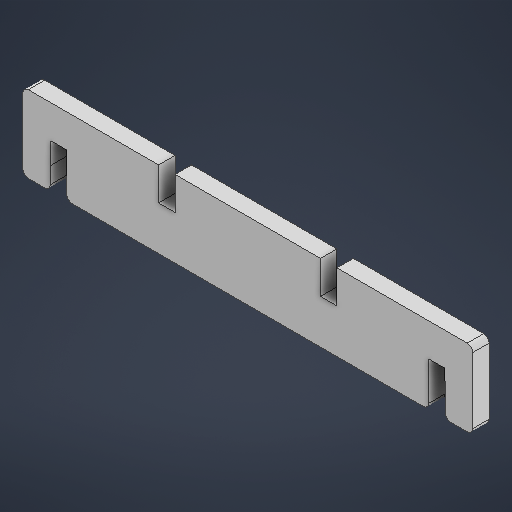
# Autodesk Inventor part: test
Saved by Autodesk Inventor 2025.3 (Build 293356030, 356C)
## iProperties
Created: 2025-10-02
Part Number: test
Material: 一般
Document SubType Name: Modeling
Designer: 陳泓任
Density: 1 g/cm^3
Appearance: 預設
Author: 陳泓任
Autodesk Inventor part; units mm, degrees
ref_plane "YZ Plane" through (0, 0, 0) normal (1, 0, 0) x (0, 1, 0)
ref_plane "XZ Plane" through (0, 0, 0) normal (0, 1, 0) x (-1, 0, 0)
ref_plane "XY Plane" through (0, 0, 0) normal (0, 0, 1) x (1, 0, 0)
sketch "草圖1" plane through (0, 0, 0) normal (0, 0, 1) x (1, 0, 0)
  line L0 (41, -6) -> (41, 6)
  line L1 (-41, 6) -> (-41, -6)
  line L2 (-40, -7) -> (-37, -7)
  line L3 (-32, -7) -> (32, -7)
  line L4 (37, -7) -> (40, -7)
  line L5 (0, 22.1211) -> (0, -32.4412) construction
  arc A0 (-40, 7) -> (-41, 6) centre (-40, 6) ccw
  arc A1 (-41, -6) -> (-40, -7) centre (-40, -6) ccw
  arc A2 (-37, -7) -> (-36, -6) centre (-37, -6) ccw
  arc A3 (-33, -6) -> (-32, -7) centre (-32, -6) ccw
  arc A4 (40, -7) -> (41, -6) centre (40, -6) ccw
  arc A5 (41, 6) -> (40, 7) centre (40, 6) ccw
  line L6 (-36, -6) -> (-36, 1) construction
  line L7 (-36, 1) -> (-33, 1) construction
  line L8 (-33, 1) -> (-33, -6)
  arc A6 (36, -6) -> (37, -7) centre (37, -6) ccw
  arc A7 (32, -7) -> (33, -6) centre (32, -6) ccw
  line L9 (36, -6) -> (36, 1) construction
  line L10 (36, 1) -> (33, 1) construction
  line L11 (33, 1) -> (33, -6)
  line L12 (-16.25, 7) -> (-16.25, 1)
  line L13 (-16.25, 1) -> (-13.25, 1)
  line L14 (-13.25, 1) -> (-13.25, 7)
  line L15 (-14.75, -1.2757) -> (-14.75, 3.2757) construction
  line L16 (16.25, 7) -> (16.25, 1)
  line L17 (16.25, 1) -> (13.25, 1)
  line L18 (13.25, 1) -> (13.25, 7)
  line L19 (-41, -7) -> (41, -7) construction
  line L20 (41, -7) -> (41, 7) construction
  line L21 (41, 7) -> (-41, 7) construction
  line L22 (-41, 7) -> (-41, -7) construction
  line L23 (-41, -7) -> (41, 7) construction
  line L24 (41, -7) -> (-41, 7) construction
  line L25 (-16.25, 7) -> (-40, 7)
  line L26 (40, 7) -> (16.25, 7)
  line L27 (13.25, 7) -> (-13.25, 7)
  line L28 (-36, -6) -> (-36, -3)
  line L29 (-35.9, 1) -> (-36, -3)
  line L30 (-35.9, 1) -> (-33, 1)
  line L31 (35.9, 1) -> (36, -3)
  line L32 (35.9, 1) -> (33, 1)
  line L33 (36, -3) -> (36, -6)
  point P0 (0, 0)
  point P1 (-14.75, 1)
  point P2 (36, -6)
  dimension "d5" = 1
  dimension "d6" = 1
  dimension "d25" = 3
  dimension "d26" = 8
  dimension "d28" = 5
  dimension "d29" = 33
  dimension "d30" = 6
  dimension "d31" = 3
  dimension "d32" = 14.75
  dimension "d34" = 14
  dimension "d35" = 4
  dimension "d36" = 0.1
  constraints: 68 end point, 17 tangent, 16 point on circle, 12 parallel, 12 perpendicular, 12 symmetric about line, 8 centre point, 8 collinear, 4 equal radius, 4 horizontal, 4 midpoint, 4 point on line, 4 vertical, 2 other
  measures "d5" radius of A0
  measures "d6" radius of A1
  measures "d25" distance of L6.end L7.end
  measures "d26" distance between parallel lines of L3 L7
  measures "d28" distance between parallel lines of L1 L6
  measures "d29" distance between parallel lines of L5 L8
  measures "d30" distance of L13.end L14.end
  measures "d31" distance of L12.end L13.end
  measures "d32" distance between parallel lines of L5 L15
  measures "d34" distance between parallel lines of L19 L21
  measures "d35" vertical distance of L28.end L29.start
  measures "d36" distance of L6.end L29.start
extrude "擠出1" add sketch "草圖1" along normal mid plane 3
